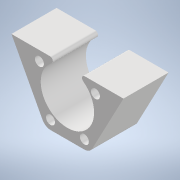
# Autodesk Inventor part: SideSpacer
Saved by Autodesk Inventor 2020 (Build 240168000, 168)
## iProperties
Created: 2020-01-23
Part Number: SideSpacer
Material: Generic
Document SubType Name: Modeling
Designer: srini
Density: 1 g/cm^3
Appearance: Default
Author: srini
Autodesk Inventor part; units mm, degrees
ref_plane "YZ Plane" through (0, 0, 0) normal (1, 0, 0) x (0, 1, 0)
ref_plane "XZ Plane" through (0, 0, 0) normal (0, 1, 0) x (-1, 0, 0)
ref_plane "XY Plane" through (0, 0, 0) normal (0, 0, 1) x (1, 0, 0)
sketch "Sketch1" plane through (0, 0, 0) normal (0, 0, 1) x (1, 0, 0)
  line L0 (-20.0409, -61.9125) -> (-18.5142, -60.3859) construction
  line L1 (-18.5142, -60.3859) -> (0, -25.4) construction
  line L2 (0, -25.4) -> (0, -2.159) construction
  line L3 (0, -2.159) -> (-2.159, 0) construction
  line L4 (-2.159, 0) -> (-61.341, 0) construction
  line L5 (-61.341, 0) -> (-63.5, -2.159) construction
  line L6 (-63.5, -2.159) -> (-63.5, -25.4) construction
  line L7 (-63.5, -25.4) -> (-44.9858, -60.3859) construction
  line L8 (-44.9858, -60.3859) -> (-43.4591, -61.9125) construction
  line L9 (-43.4591, -61.9125) -> (-20.0409, -61.9125) construction
  circle A0 centre (-22.225, -57.0353) radius 2.0701 construction
  circle A1 centre (-47.5103, -31.75) radius 2.0701 construction
  circle A2 centre (-31.75, -12.7) radius 2.0701 construction
  circle A3 centre (-6.35, -12.7) radius 2.0701 construction
  circle A4 centre (-31.75, -41.275) radius 14.2875 construction
  circle A5 centre (-57.15, -12.7) radius 2.0701 construction
  circle A6 centre (-44.45, -12.7) radius 2.0701 construction
  circle A7 centre (-19.05, -12.7) radius 2.0701 construction
  circle A8 centre (-41.275, -57.0353) radius 2.0701 construction
  circle A9 centre (-15.9897, -31.75) radius 2.0701 construction
  circle A10 centre (-47.5103, -31.75) radius 2.54
  circle A11 centre (-15.9897, -31.75) radius 2.54
  circle A12 centre (-41.275, -57.0353) radius 2.54
  circle A13 centre (-22.225, -57.0353) radius 2.54
  circle A14 centre (-47.5103, -31.75) radius 3.4
  arc A15 (-42.1702, -52.0856) -> (-36.4766, -55.5267) centre (-41.275, -57.0353) ccw
  line L10 (-63.2519, -26.26) -> (-44.3041, -62.0653)
  line L11 (-44.3041, -62.0653) -> (-19.1959, -62.0653)
  line L12 (-19.1959, -62.0653) -> (-0.2481, -26.26)
  line L13 (-0.2481, -26.26) -> (-21.9855, -26.26)
  arc A16 (-27.0234, -55.5267) -> (-21.3298, -52.0856) centre (-22.225, -57.0353) ccw
  arc A17 (-36.4766, -55.5267) -> (-27.0234, -55.5267) centre (-31.75, -41.275) ccw
  arc A18 (-42.1702, -52.0856) -> (-36.4766, -55.5267) centre (-31.75, -41.275) ccw
  arc A19 (-27.0234, -55.5267) -> (-21.3298, -52.0856) centre (-31.75, -41.275) ccw
  arc A20 (-21.3298, -52.0856) -> (-22.9192, -29.1314) centre (-31.75, -41.275) ccw
  arc A21 (-41.1827, -52.0061) -> (-42.1702, -52.0856) centre (-41.275, -57.0353) ccw
  arc A22 (-36.8654, -54.6154) -> (-41.1827, -52.0061) centre (-41.275, -57.0353) ccw construction
  arc A23 (-26.6346, -54.6154) -> (-27.0234, -55.5267) centre (-22.225, -57.0353) ccw
  arc A24 (-22.3173, -52.0061) -> (-26.6346, -54.6154) centre (-22.225, -57.0353) ccw construction
  arc A25 (-36.4766, -55.5267) -> (-36.8654, -54.6154) centre (-41.275, -57.0353) ccw
  arc A26 (-21.3298, -52.0856) -> (-22.3173, -52.0061) centre (-22.225, -57.0353) ccw
  line L14 (450.85, -25.4) -> (-107.95, -25.4) projected
  line L15 (-41.5145, -26.26) -> (-63.2519, -26.26)
  arc A27 (-40.5808, -29.1314) -> (-42.1702, -52.0856) centre (-31.75, -41.275) ccw
  arc A28 (-40.5808, -29.1314) -> (-41.5145, -26.26) centre (-41.5145, -27.8475) ccw
  arc A29 (-21.9855, -26.26) -> (-22.9192, -29.1314) centre (-21.9855, -27.8475) ccw
  point P0 (0, 0)
  point P1 (-44.6004, -33.5086)
  point P2 (-31.75, -26.26)
  point P3 (-45.7209, -59.388)
  point P4 (-41.275, -62.0653)
  point P5 (-22.225, -62.0653)
  point P6 (-17.7791, -59.388)
  point P7 (-31.75, -26.26)
  point P8 (-44.6004, -33.5086)
  dimension "d0" = 5.08
  dimension "d1" = 6.8
  dimension "d2" = 10.06
  dimension "d8" = 1.5875
  constraints: 38 point on circle, 21 tangent, 20 centre point, 10 end point, 8 coincident, 5 equal radius, 2 horizontal, 2 point on line, 1 equal length, 1 parallel
  measures "d0" diameter of A10
  measures "d1" diameter of A14
  measures "d2" diameter of A15
  measures "d8" radius of A28
extrude "Extrusion1" add sketch "Sketch1" along normal blind 25.4 contours A14 | A27 A15 L10 L15 A28 | A18 A15 | A17 A16 L11 A15 | A19 A16 | A20 A29 L13 L12 A16
body "Solid1"
